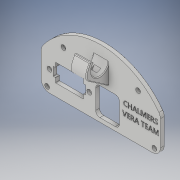
# Autodesk Inventor part: AdapterChassiContact
Saved by Autodesk Inventor 2019.3 (Build 233278000, 278)
## iProperties
Created: 2019-02-24
Part Number: AdapterChassiContact
Material: Generic
Document SubType Name: Modeling
Designer: Johansson
Density: 1 g/cm^3
Appearance: Default
Author: Johansson
## iProperties of the stored document AdapterChassiContact_3DPrint.ipt
Created: 2019-02-24
Part Number: AdapterChassiContact_3DPrint
Material: Generic
Document SubType Name: Modeling
Designer: Johansson
Density: 1 g/cm^3
Appearance: Default
Author: Johansson
Autodesk Inventor part; units mm, degrees
(part 1 of 4)
ref_plane "YZ Plane" through (0, 0, 0) normal (1, 0, 0) x (0, 1, 0)
ref_plane "XZ Plane" through (0, 0, 0) normal (0, 1, 0) x (-1, 0, 0)
ref_plane "XY Plane" through (0, 0, 0) normal (0, 0, 1) x (1, 0, 0)
sketch "Sketch1" plane through (0, 0, 0) normal (0, 0, 1) x (1, 0, 0)
  line L0 (-75, -22.5) -> (75, -22.5)
  line L1 (75, -22.5) -> (75, 22.5)
  line L2 (75, 22.5) -> (-75, 22.5)
  line L3 (-75, 22.5) -> (-75, -22.5)
  line L4 (-75, -22.5) -> (75, 22.5) construction
  line L5 (75, -22.5) -> (-75, 22.5) construction
  arc A0 (75, 22.5) -> (-75, 22.5) centre (0, -27.8125) ccw
  point P0 (0, 0)
  dimension "d0" = 150
  dimension "d1" = 85
  dimension "d2" = 45
  constraints: 12 end point, 2 midpoint, 2 parallel, 2 point on circle, 1 centre point, 1 horizontal, 1 perpendicular
  measures "d0" distance of L0.start L0.end
  measures "d1" distance edge to line of A0 L0
  measures "d2" distance of L0.end L1.end
extrude "Extrusion1" add sketch "Sketch1" along normal blind 5
sketch "Sketch2" plane through (0, 0, 5) normal (0, 0, 1) x (1, 0, 0)
  spline S0 degree 3 poles (-2.5291, 34.9419) (-3.1837, 35.0019) (-3.8439, 35.3955) (-4.2067, 35.9422) knots 0 0 0 0 1 1 1 1
  line L0 (-2.5291, 34.9419) -> (-3.1837, 35.0019) construction
  line L1 (-3.1837, 35.0019) -> (-3.8439, 35.3955) construction
  line L2 (-3.8439, 35.3955) -> (-4.2067, 35.9422) construction
  spline S1 degree 3 poles (-4.2067, 35.9422) (-4.5423, 36.4477) (-4.6869, 37.074) (-4.5949, 37.6226) knots 1 1 1 1 2 2 2 2
  line L3 (-4.2067, 35.9422) -> (-4.5423, 36.4477) construction
  line L4 (-4.5423, 36.4477) -> (-4.6869, 37.074) construction
  line L5 (-4.6869, 37.074) -> (-4.5949, 37.6226) construction
  spline S2 degree 3 poles (-4.5949, 37.6226) (-4.5028, 38.1713) (-4.29, 38.5913) (-3.9153, 38.9637) knots 2 2 2 2 3 3 3 3
  line L6 (-4.5949, 37.6226) -> (-4.5028, 38.1713) construction
  line L7 (-4.5028, 38.1713) -> (-4.29, 38.5913) construction
  line L8 (-4.29, 38.5913) -> (-3.9153, 38.9637) construction
  spline S3 degree 3 poles (-3.9153, 38.9637) (-3.6201, 39.257) (-3.2509, 39.4631) (-2.8284, 39.5702) knots 3 3 3 3 4 4 4 4
  line L9 (-3.9153, 38.9637) -> (-3.6201, 39.257) construction
  line L10 (-3.6201, 39.257) -> (-3.2509, 39.4631) construction
  line L11 (-3.2509, 39.4631) -> (-2.8284, 39.5702) construction
  spline S4 degree 3 poles (-2.8284, 39.5702) (-2.5997, 39.6282) (-2.3286, 39.6529) (-2.1379, 39.6331) knots 4 4 4 4 5 5 5 5
  line L12 (-2.8284, 39.5702) -> (-2.5997, 39.6282) construction
  line L13 (-2.5997, 39.6282) -> (-2.3286, 39.6529) construction
  line L14 (-2.3286, 39.6529) -> (-2.1379, 39.6331) construction
  spline S5 degree 3 poles (-2.1379, 39.6331) (-1.8898, 39.6073) (-1.8541, 39.6014) (-1.7115, 39.563) knots 5 5 5 5 6 6 6 6
  line L15 (-2.1379, 39.6331) -> (-1.8898, 39.6073) construction
  line L16 (-1.8898, 39.6073) -> (-1.8541, 39.6014) construction
  line L17 (-1.8541, 39.6014) -> (-1.7115, 39.563) construction
  spline S6 degree 3 poles (-1.7115, 39.563) (-1.5406, 39.517) (-1.5075, 39.5031) (-0.386, 39.0072) knots 6 6 6 6 7 7 7 7
  line L18 (-1.7115, 39.563) -> (-1.5406, 39.517) construction
  line L19 (-1.5406, 39.517) -> (-1.5075, 39.5031) construction
  line L20 (-1.5075, 39.5031) -> (-0.386, 39.0072) construction
  spline S7 degree 3 poles (-0.386, 39.0072) (0.5004, 38.6152) (0.8357, 38.4674) (0.9545, 38.4164) knots 7 7 7 7 8 8 8 8
  line L21 (-0.386, 39.0072) -> (0.5004, 38.6152) construction
  line L22 (0.5004, 38.6152) -> (0.8357, 38.4674) construction
  line L23 (0.8357, 38.4674) -> (0.9545, 38.4164) construction
  spline S8 degree 3 poles (0.9545, 38.4164) (1.1108, 38.3493) (1.1389, 38.3282) (1.072, 38.3282) (1.0454, 38.3282) (0.9942, 38.3132) (0.9582, 38.2948) knots 8 8 8 8 9 9 9 10 10 10 10
  line L24 (0.9545, 38.4164) -> (1.1108, 38.3493) construction
  line L25 (1.1108, 38.3493) -> (1.1389, 38.3282) construction
  line L26 (1.1389, 38.3282) -> (1.072, 38.3282) construction
  line L27 (1.072, 38.3282) -> (1.0454, 38.3282) construction
  line L28 (1.0454, 38.3282) -> (0.9942, 38.3132) construction
  line L29 (0.9942, 38.3132) -> (0.9582, 38.2948) construction
  line L30 (0.9582, 38.2948) -> (0.8926, 38.2613)
  line L31 (0.8926, 38.2613) -> (0.2754, 38.5244)
  spline S9 degree 3 poles (0.2754, 38.5244) (-0.0641, 38.6691) (-0.4798, 38.8468) (-0.6484, 38.9191) (-0.817, 38.9915) (-0.9608, 39.0471) (-0.968, 39.0426) knots 12 12 12 12 13 13 13 14 14 14 14
  line L32 (0.2754, 38.5244) -> (-0.0641, 38.6691) construction
  line L33 (-0.0641, 38.6691) -> (-0.4798, 38.8468) construction
  line L34 (-0.4798, 38.8468) -> (-0.6484, 38.9191) construction
  line L35 (-0.6484, 38.9191) -> (-0.817, 38.9915) construction
  line L36 (-0.817, 38.9915) -> (-0.9608, 39.0471) construction
  line L37 (-0.9608, 39.0471) -> (-0.968, 39.0426) construction
  spline S10 degree 3 poles (-0.968, 39.0426) (-0.9926, 39.0275) (-1.0039, 38.9233) (-0.9836, 38.899) knots 14 14 14 14 15 15 15 15
  line L38 (-0.968, 39.0426) -> (-0.9926, 39.0275) construction
  line L39 (-0.9926, 39.0275) -> (-1.0039, 38.9233) construction
  line L40 (-1.0039, 38.9233) -> (-0.9836, 38.899) construction
  spline S11 degree 3 poles (-0.9836, 38.899) (-0.9576, 38.8675) (-0.8953, 38.8685) (-0.8524, 38.9009) knots 15 15 15 15 16 16 16 16
  line L41 (-0.9836, 38.899) -> (-0.9576, 38.8675) construction
  line L42 (-0.9576, 38.8675) -> (-0.8953, 38.8685) construction
  line L43 (-0.8953, 38.8685) -> (-0.8524, 38.9009) construction
  spline S12 degree 3 poles (-0.8524, 38.9009) (-0.7927, 38.9461) (-0.7695, 38.935) (-0.8001, 38.8759) knots 16 16 16 16 17 17 17 17
  line L44 (-0.8524, 38.9009) -> (-0.7927, 38.9461) construction
  line L45 (-0.7927, 38.9461) -> (-0.7695, 38.935) construction
  line L46 (-0.7695, 38.935) -> (-0.8001, 38.8759) construction
  spline S13 degree 3 poles (-0.8001, 38.8759) (-0.8345, 38.8092) (-0.8342, 38.7619) (-0.7991, 38.7328) knots 17 17 17 17 18 18 18 18
  line L47 (-0.8001, 38.8759) -> (-0.8345, 38.8092) construction
  line L48 (-0.8345, 38.8092) -> (-0.8342, 38.7619) construction
  line L49 (-0.8342, 38.7619) -> (-0.7991, 38.7328) construction
  spline S14 degree 3 poles (-0.7991, 38.7328) (-0.7761, 38.7136) (-0.758, 38.7146) (-0.6933, 38.7386) knots 18 18 18 18 19 19 19 19
  line L50 (-0.7991, 38.7328) -> (-0.7761, 38.7136) construction
  line L51 (-0.7761, 38.7136) -> (-0.758, 38.7146) construction
  line L52 (-0.758, 38.7146) -> (-0.6933, 38.7386) construction
  spline S15 degree 3 poles (-0.6933, 38.7386) (-0.6055, 38.7711) (-0.6012, 38.766) (-0.6497, 38.6865) knots 19 19 19 19 20 20 20 20
  line L53 (-0.6933, 38.7386) -> (-0.6055, 38.7711) construction
  line L54 (-0.6055, 38.7711) -> (-0.6012, 38.766) construction
  line L55 (-0.6012, 38.766) -> (-0.6497, 38.6865) construction
  spline S16 degree 3 poles (-0.6497, 38.6865) (-0.6836, 38.6309) (-0.6836, 38.63) (-0.6495, 38.5866) knots 20 20 20 20 21 21 21 21
  line L56 (-0.6497, 38.6865) -> (-0.6836, 38.6309) construction
  line L57 (-0.6836, 38.6309) -> (-0.6836, 38.63) construction
  line L58 (-0.6836, 38.63) -> (-0.6495, 38.5866) construction
  spline S17 degree 3 poles (-0.6495, 38.5866) (-0.6157, 38.5436) (-0.6137, 38.5433) (-0.5444, 38.5706) knots 21 21 21 21 22 22 22 22
  line L59 (-0.6495, 38.5866) -> (-0.6157, 38.5436) construction
  line L60 (-0.6157, 38.5436) -> (-0.6137, 38.5433) construction
  line L61 (-0.6137, 38.5433) -> (-0.5444, 38.5706) construction
  spline S18 degree 3 poles (-0.5444, 38.5706) (-0.5056, 38.5858) (-0.4691, 38.5936) (-0.4634, 38.5879) knots 22 22 22 22 23 23 23 23
  line L62 (-0.5444, 38.5706) -> (-0.5056, 38.5858) construction
  line L63 (-0.5056, 38.5858) -> (-0.4691, 38.5936) construction
  line L64 (-0.4691, 38.5936) -> (-0.4634, 38.5879) construction
  spline S19 degree 3 poles (-0.4634, 38.5879) (-0.4577, 38.5822) (-0.4736, 38.5504) (-0.4989, 38.5173) knots 23 23 23 23 24 24 24 24
  line L65 (-0.4634, 38.5879) -> (-0.4577, 38.5822) construction
  line L66 (-0.4577, 38.5822) -> (-0.4736, 38.5504) construction
  line L67 (-0.4736, 38.5504) -> (-0.4989, 38.5173) construction
  spline S20 degree 3 poles (-0.4989, 38.5173) (-0.552, 38.4477) (-0.5549, 38.4291) (-0.5176, 38.3982) knots 24 24 24 24 25 25 25 25
  line L68 (-0.4989, 38.5173) -> (-0.552, 38.4477) construction
  line L69 (-0.552, 38.4477) -> (-0.5549, 38.4291) construction
  line L70 (-0.5549, 38.4291) -> (-0.5176, 38.3982) construction
  spline S21 degree 3 poles (-0.5176, 38.3982) (-0.4964, 38.3806) (-0.476, 38.3801) (-0.4254, 38.3956) knots 25 25 25 25 26 26 26 26
  line L71 (-0.5176, 38.3982) -> (-0.4964, 38.3806) construction
  line L72 (-0.4964, 38.3806) -> (-0.476, 38.3801) construction
  line L73 (-0.476, 38.3801) -> (-0.4254, 38.3956) construction
  spline S22 degree 3 poles (-0.4254, 38.3956) (-0.3345, 38.4235) (-0.3128, 38.3954) (-0.3752, 38.3302) knots 26 26 26 26 27 27 27 27
  line L74 (-0.4254, 38.3956) -> (-0.3345, 38.4235) construction
  line L75 (-0.3345, 38.4235) -> (-0.3128, 38.3954) construction
  line L76 (-0.3128, 38.3954) -> (-0.3752, 38.3302) construction
  spline S23 degree 3 poles (-0.3752, 38.3302) (-0.4071, 38.297) (-0.4222, 38.2646) (-0.4183, 38.2375) knots 27 27 27 27 28 28 28 28
  line L77 (-0.3752, 38.3302) -> (-0.4071, 38.297) construction
  line L78 (-0.4071, 38.297) -> (-0.4222, 38.2646) construction
  line L79 (-0.4222, 38.2646) -> (-0.4183, 38.2375) construction
  spline S24 degree 3 poles (-0.4183, 38.2375) (-0.4129, 38.199) (-0.4056, 38.1963) (-0.3198, 38.2016) knots 28 28 28 28 29 29 29 29
  line L80 (-0.4183, 38.2375) -> (-0.4129, 38.199) construction
  line L81 (-0.4129, 38.199) -> (-0.4056, 38.1963) construction
  line L82 (-0.4056, 38.1963) -> (-0.3198, 38.2016) construction
  spline S25 degree 3 poles (-0.3198, 38.2016) (-0.2689, 38.2047) (-0.2272, 38.2011) (-0.2272, 38.1936) (-0.2272, 38.1861) (-0.2524, 38.154) (-0.2832, 38.1222) knots 29 29 29 29 30 30 30 31 31 31 31
  line L83 (-0.3198, 38.2016) -> (-0.2689, 38.2047) construction
  line L84 (-0.2689, 38.2047) -> (-0.2272, 38.2011) construction
  line L85 (-0.2272, 38.2011) -> (-0.2272, 38.1936) construction
  line L86 (-0.2272, 38.1936) -> (-0.2272, 38.1861) construction
  line L87 (-0.2272, 38.1861) -> (-0.2524, 38.154) construction
  line L88 (-0.2524, 38.154) -> (-0.2832, 38.1222) construction
  spline S26 degree 3 poles (-0.2832, 38.1222) (-0.333, 38.0708) (-0.3369, 38.0596) (-0.3188, 38.02) knots 31 31 31 31 32 32 32 32
  line L89 (-0.2832, 38.1222) -> (-0.333, 38.0708) construction
  line L90 (-0.333, 38.0708) -> (-0.3369, 38.0596) construction
  line L91 (-0.3369, 38.0596) -> (-0.3188, 38.02) construction
  spline S27 degree 3 poles (-0.3188, 38.02) (-0.3014, 37.9816) (-0.287, 37.9753) (-0.2144, 37.9748) knots 32 32 32 32 33 33 33 33
  line L92 (-0.3188, 38.02) -> (-0.3014, 37.9816) construction
  line L93 (-0.3014, 37.9816) -> (-0.287, 37.9753) construction
  line L94 (-0.287, 37.9753) -> (-0.2144, 37.9748) construction
  line L95 (-0.2144, 37.9748) -> (-0.1302, 37.9741)
  line L96 (-0.1302, 37.9741) -> (-0.1964, 37.9174)
  spline S28 degree 3 poles (-0.1964, 37.9174) (-0.2328, 37.8863) (-0.2625, 37.8472) (-0.2625, 37.8305) (-0.2625, 37.7908) (-0.2095, 37.7638) (-0.1314, 37.7638) (-0.0518, 37.7638) (-0.0515, 37.742) (-0.1307, 37.6953) knots 35 35 35 35 36 36 36 37 37 37 38 38 38 38
  line L97 (-0.1964, 37.9174) -> (-0.2328, 37.8863) construction
  line L98 (-0.2328, 37.8863) -> (-0.2625, 37.8472) construction
  line L99 (-0.2625, 37.8472) -> (-0.2625, 37.8305) construction
  line L100 (-0.2625, 37.8305) -> (-0.2625, 37.7908) construction
  line L101 (-0.2625, 37.7908) -> (-0.2095, 37.7638) construction
  line L102 (-0.2095, 37.7638) -> (-0.1314, 37.7638) construction
  line L103 (-0.1314, 37.7638) -> (-0.0518, 37.7638) construction
  line L104 (-0.0518, 37.7638) -> (-0.0515, 37.742) construction
  line L105 (-0.0515, 37.742) -> (-0.1307, 37.6953) construction
  spline S29 degree 3 poles (-0.1307, 37.6953) (-0.2375, 37.6322) (-0.2296, 37.5664) (-0.1126, 37.5444) knots 38 38 38 38 39 39 39 39
  line L106 (-0.1307, 37.6953) -> (-0.2375, 37.6322) construction
  line L107 (-0.2375, 37.6322) -> (-0.2296, 37.5664) construction
  line L108 (-0.2296, 37.5664) -> (-0.1126, 37.5444) construction
  spline S30 degree 3 poles (-0.1126, 37.5444) (-0.025, 37.528) (-0.0224, 37.5054) (-0.1032, 37.4642) knots 39 39 39 39 40 40 40 40
  line L109 (-0.1126, 37.5444) -> (-0.025, 37.528) construction
  line L110 (-0.025, 37.528) -> (-0.0224, 37.5054) construction
  line L111 (-0.0224, 37.5054) -> (-0.1032, 37.4642) construction
  spline S31 degree 3 poles (-0.1032, 37.4642) (-0.1559, 37.4373) (-0.1743, 37.4171) (-0.1743, 37.3863) (-0.1743, 37.3358) (-0.1496, 37.3136) (-0.0685, 37.2914) knots 40 40 40 40 41 41 41 42 42 42 42
  line L112 (-0.1032, 37.4642) -> (-0.1559, 37.4373) construction
  line L113 (-0.1559, 37.4373) -> (-0.1743, 37.4171) construction
  line L114 (-0.1743, 37.4171) -> (-0.1743, 37.3863) construction
  line L115 (-0.1743, 37.3863) -> (-0.1743, 37.3358) construction
  line L116 (-0.1743, 37.3358) -> (-0.1496, 37.3136) construction
  line L117 (-0.1496, 37.3136) -> (-0.0685, 37.2914) construction
  line L118 (-0.0685, 37.2914) -> (-0.0068, 37.2745)
  line L119 (-0.0068, 37.2745) -> (-0.0597, 37.2545)
  spline S32 degree 3 poles (-0.0597, 37.2545) (-0.1458, 37.2221) (-0.1652, 37.2067) (-0.1713, 37.1657) knots 44 44 44 44 45 45 45 45
  line L120 (-0.0597, 37.2545) -> (-0.1458, 37.2221) construction
  line L121 (-0.1458, 37.2221) -> (-0.1652, 37.2067) construction
  line L122 (-0.1652, 37.2067) -> (-0.1713, 37.1657) construction
  spline S33 degree 3 poles (-0.1713, 37.1657) (-0.1788, 37.115) (-0.149, 37.0808) (-0.0849, 37.0668) knots 45 45 45 45 46 46 46 46
  line L123 (-0.1713, 37.1657) -> (-0.1788, 37.115) construction
  line L124 (-0.1788, 37.115) -> (-0.149, 37.0808) construction
  line L125 (-0.149, 37.0808) -> (-0.0849, 37.0668) construction
  spline S34 degree 3 poles (-0.0849, 37.0668) (-0.0168, 37.0518) (-0.0193, 37.0287) (-0.0905, 37.0135) knots 46 46 46 46 47 47 47 47
  line L126 (-0.0849, 37.0668) -> (-0.0168, 37.0518) construction
  line L127 (-0.0168, 37.0518) -> (-0.0193, 37.0287) construction
  line L128 (-0.0193, 37.0287) -> (-0.0905, 37.0135) construction
  spline S35 degree 3 poles (-0.0905, 37.0135) (-0.1665, 36.9972) (-0.192, 36.9746) (-0.192, 36.9232) (-0.192, 36.8928) (-0.1732, 36.8696) (-0.1264, 36.8419) knots 47 47 47 47 48 48 48 49 49 49 49
  line L129 (-0.0905, 37.0135) -> (-0.1665, 36.9972) construction
  line L130 (-0.1665, 36.9972) -> (-0.192, 36.9746) construction
  line L131 (-0.192, 36.9746) -> (-0.192, 36.9232) construction
  line L132 (-0.192, 36.9232) -> (-0.192, 36.8928) construction
  line L133 (-0.192, 36.8928) -> (-0.1732, 36.8696) construction
  line L134 (-0.1732, 36.8696) -> (-0.1264, 36.8419) construction
  line L135 (-0.1264, 36.8419) -> (-0.0608, 36.8032)
  line L136 (-0.0608, 36.8032) -> (-0.1355, 36.7905)
  spline S36 degree 3 poles (-0.1355, 36.7905) (-0.2322, 36.774) (-0.2449, 36.765) (-0.2449, 36.7134) (-0.2449, 36.6838) (-0.2258, 36.6581) (-0.1834, 36.6306) knots 51 51 51 51 52 52 52 53 53 53 53
  line L137 (-0.1355, 36.7905) -> (-0.2322, 36.774) construction
  line L138 (-0.2322, 36.774) -> (-0.2449, 36.765) construction
  line L139 (-0.2449, 36.765) -> (-0.2449, 36.7134) construction
  line L140 (-0.2449, 36.7134) -> (-0.2449, 36.6838) construction
  line L141 (-0.2449, 36.6838) -> (-0.2258, 36.6581) construction
  line L142 (-0.2258, 36.6581) -> (-0.1834, 36.6306) construction
  spline S37 degree 3 poles (-0.1834, 36.6306) (-0.1495, 36.6087) (-0.1218, 36.5848) (-0.1216, 36.5775) knots 53 53 53 53 54 54 54 54
  line L143 (-0.1834, 36.6306) -> (-0.1495, 36.6087) construction
  line L144 (-0.1495, 36.6087) -> (-0.1218, 36.5848) construction
  line L145 (-0.1218, 36.5848) -> (-0.1216, 36.5775) construction
  spline S38 degree 3 poles (-0.1216, 36.5775) (-0.1215, 36.5703) (-0.1573, 36.5643) (-0.2012, 36.5643) (-0.2693, 36.5643) (-0.2839, 36.5578) (-0.3012, 36.5198) knots 54 54 54 54 55 55 55 56 56 56 56
  line L146 (-0.1216, 36.5775) -> (-0.1215, 36.5703) construction
  line L147 (-0.1215, 36.5703) -> (-0.1573, 36.5643) construction
  line L148 (-0.1573, 36.5643) -> (-0.2012, 36.5643) construction
  line L149 (-0.2012, 36.5643) -> (-0.2693, 36.5643) construction
  line L150 (-0.2693, 36.5643) -> (-0.2839, 36.5578) construction
  line L151 (-0.2839, 36.5578) -> (-0.3012, 36.5198) construction
  spline S39 degree 3 poles (-0.3012, 36.5198) (-0.3194, 36.4799) (-0.3153, 36.4688) (-0.2621, 36.414) knots 56 56 56 56 57 57 57 57
  line L152 (-0.3012, 36.5198) -> (-0.3194, 36.4799) construction
  line L153 (-0.3194, 36.4799) -> (-0.3153, 36.4688) construction
  line L154 (-0.3153, 36.4688) -> (-0.2621, 36.414) construction
  line L155 (-0.2621, 36.414) -> (-0.2027, 36.3526)
  line L156 (-0.2027, 36.3526) -> (-0.282, 36.3526)
  spline S40 degree 3 poles (-0.282, 36.3526) (-0.4153, 36.3526) (-0.4392, 36.2947) (-0.3463, 36.1971) knots 59 59 59 59 60 60 60 60
  line L157 (-0.282, 36.3526) -> (-0.4153, 36.3526) construction
  line L158 (-0.4153, 36.3526) -> (-0.4392, 36.2947) construction
  line L159 (-0.4392, 36.2947) -> (-0.3463, 36.1971) construction
  line L160 (-0.3463, 36.1971) -> (-0.289, 36.1368)
  line L161 (-0.289, 36.1368) -> (-0.3739, 36.1489)
  spline S41 degree 3 poles (-0.3739, 36.1489) (-0.5046, 36.1677) (-0.5488, 36.1076) (-0.4742, 36.0127) knots 62 62 62 62 63 63 63 63
  line L162 (-0.3739, 36.1489) -> (-0.5046, 36.1677) construction
  line L163 (-0.5046, 36.1677) -> (-0.5488, 36.1076) construction
  line L164 (-0.5488, 36.1076) -> (-0.4742, 36.0127) construction
  spline S42 degree 3 poles (-0.4742, 36.0127) (-0.4548, 35.988) (-0.4389, 35.9623) (-0.4389, 35.9555) (-0.4389, 35.9436) (-0.4945, 35.9532) (-0.5506, 35.9747) knots 63 63 63 63 64 64 64 65 65 65 65
  line L165 (-0.4742, 36.0127) -> (-0.4548, 35.988) construction
  line L166 (-0.4548, 35.988) -> (-0.4389, 35.9623) construction
  line L167 (-0.4389, 35.9623) -> (-0.4389, 35.9555) construction
  line L168 (-0.4389, 35.9555) -> (-0.4389, 35.9436) construction
  line L169 (-0.4389, 35.9436) -> (-0.4945, 35.9532) construction
  line L170 (-0.4945, 35.9532) -> (-0.5506, 35.9747) construction
  spline S43 degree 3 poles (-0.5506, 35.9747) (-0.5654, 35.9804) (-0.5937, 35.9686) (-0.6142, 35.9481) knots 65 65 65 65 66 66 66 66
  line L171 (-0.5506, 35.9747) -> (-0.5654, 35.9804) construction
  line L172 (-0.5654, 35.9804) -> (-0.5937, 35.9686) construction
  line L173 (-0.5937, 35.9686) -> (-0.6142, 35.9481) construction
  line L174 (-0.6142, 35.9481) -> (-0.6511, 35.9112)
  line L175 (-0.6511, 35.9112) -> (-0.6155, 35.8416)
  spline S44 degree 3 poles (-0.6155, 35.8416) (-0.5691, 35.7506) (-0.5702, 35.7469) (-0.6341, 35.78) knots 68 68 68 68 69 69 69 69
  line L176 (-0.6155, 35.8416) -> (-0.5691, 35.7506) construction
  line L177 (-0.5691, 35.7506) -> (-0.5702, 35.7469) construction
  line L178 (-0.5702, 35.7469) -> (-0.6341, 35.78) construction
  spline S45 degree 3 poles (-0.6341, 35.78) (-0.6987, 35.8134) (-0.7546, 35.8083) (-0.7807, 35.7666) knots 69 69 69 69 70 70 70 70
  line L179 (-0.6341, 35.78) -> (-0.6987, 35.8134) construction
  line L180 (-0.6987, 35.8134) -> (-0.7546, 35.8083) construction
  line L181 (-0.7546, 35.8083) -> (-0.7807, 35.7666) construction
  spline S46 degree 3 poles (-0.7807, 35.7666) (-0.7994, 35.7368) (-0.7973, 35.7265) (-0.7466, 35.604) knots 70 70 70 70 71 71 71 71
  line L182 (-0.7807, 35.7666) -> (-0.7994, 35.7368) construction
  line L183 (-0.7994, 35.7368) -> (-0.7973, 35.7265) construction
  line L184 (-0.7973, 35.7265) -> (-0.7466, 35.604) construction
  spline S47 degree 3 poles (-0.7466, 35.604) (-0.7333, 35.572) (-0.7367, 35.5724) (-0.797, 35.6097) knots 71 71 71 71 72 72 72 72
  line L185 (-0.7466, 35.604) -> (-0.7333, 35.572) construction
  line L186 (-0.7333, 35.572) -> (-0.7367, 35.5724) construction
  line L187 (-0.7367, 35.5724) -> (-0.797, 35.6097) construction
  spline S48 degree 3 poles (-0.797, 35.6097) (-0.889, 35.6665) (-0.9404, 35.6551) (-0.9462, 35.5765) knots 72 72 72 72 73 73 73 73
  line L188 (-0.797, 35.6097) -> (-0.889, 35.6665) construction
  line L189 (-0.889, 35.6665) -> (-0.9404, 35.6551) construction
  line L190 (-0.9404, 35.6551) -> (-0.9462, 35.5765) construction
  spline S49 degree 3 poles (-0.9462, 35.5765) (-0.9554, 35.4536) (-0.9433, 35.4538) (-0.6443, 35.5823) knots 73 73 73 73 74 74 74 74
  line L191 (-0.9462, 35.5765) -> (-0.9554, 35.4536) construction
  line L192 (-0.9554, 35.4536) -> (-0.9433, 35.4538) construction
  line L193 (-0.9433, 35.4538) -> (-0.6443, 35.5823) construction
  spline S50 degree 3 poles (-0.6443, 35.5823) (-0.4937, 35.647) (-0.3654, 35.7) (-0.3592, 35.7) (-0.353, 35.7) (-0.2196, 35.7549) (-0.0627, 35.8219) knots 74 74 74 74 75 75 75 76 76 76 76
  line L194 (-0.6443, 35.5823) -> (-0.4937, 35.647) construction
  line L195 (-0.4937, 35.647) -> (-0.3654, 35.7) construction
  line L196 (-0.3654, 35.7) -> (-0.3592, 35.7) construction
  line L197 (-0.3592, 35.7) -> (-0.353, 35.7) construction
  line L198 (-0.353, 35.7) -> (-0.2196, 35.7549) construction
  line L199 (-0.2196, 35.7549) -> (-0.0627, 35.8219) construction
  spline S51 degree 3 poles (-0.0627, 35.8219) (0.0942, 35.889) (0.337, 35.9927) (0.4769, 36.0523) knots 76 76 76 76 77 77 77 77
  line L200 (-0.0627, 35.8219) -> (0.0942, 35.889) construction
  line L201 (0.0942, 35.889) -> (0.337, 35.9927) construction
  line L202 (0.337, 35.9927) -> (0.4769, 36.0523) construction
  spline S52 degree 3 poles (0.4769, 36.0523) (0.6168, 36.112) (0.7546, 36.1729) (0.783, 36.1876) knots 77 77 77 77 78 78 78 78
  line L203 (0.4769, 36.0523) -> (0.6168, 36.112) construction
  line L204 (0.6168, 36.112) -> (0.7546, 36.1729) construction
  line L205 (0.7546, 36.1729) -> (0.783, 36.1876) construction
  spline S53 degree 3 poles (0.783, 36.1876) (0.833, 36.2134) (0.8367, 36.2125) (0.8866, 36.1615) knots 78 78 78 78 79 79 79 79
  line L206 (0.783, 36.1876) -> (0.833, 36.2134) construction
  line L207 (0.833, 36.2134) -> (0.8367, 36.2125) construction
  line L208 (0.8367, 36.2125) -> (0.8866, 36.1615) construction
  spline S54 degree 3 poles (0.8866, 36.1615) (0.915, 36.1324) (0.932, 36.1049) (0.9244, 36.1003) knots 79 79 79 79 80 80 80 80
  line L209 (0.8866, 36.1615) -> (0.915, 36.1324) construction
  line L210 (0.915, 36.1324) -> (0.932, 36.1049) construction
  line L211 (0.932, 36.1049) -> (0.9244, 36.1003) construction
  spline S55 degree 3 poles (0.9244, 36.1003) (0.9167, 36.0958) (0.7795, 36.0389) (0.6194, 35.9738) knots 80 80 80 80 81 81 81 81
  line L212 (0.9244, 36.1003) -> (0.9167, 36.0958) construction
  line L213 (0.9167, 36.0958) -> (0.7795, 36.0389) construction
  line L214 (0.7795, 36.0389) -> (0.6194, 35.9738) construction
  spline S56 degree 3 poles (0.6194, 35.9738) (0.4593, 35.9087) (0.3204, 35.8495) (0.3107, 35.8422) knots 81 81 81 81 82 82 82 82
  line L215 (0.6194, 35.9738) -> (0.4593, 35.9087) construction
  line L216 (0.4593, 35.9087) -> (0.3204, 35.8495) construction
  line L217 (0.3204, 35.8495) -> (0.3107, 35.8422) construction
  spline S57 degree 3 poles (0.3107, 35.8422) (0.301, 35.8348) (0.2296, 35.8028) (0.152, 35.7711) knots 82 82 82 82 83 83 83 83
  line L218 (0.3107, 35.8422) -> (0.301, 35.8348) construction
  line L219 (0.301, 35.8348) -> (0.2296, 35.8028) construction
  line L220 (0.2296, 35.8028) -> (0.152, 35.7711) construction
  spline S58 degree 3 poles (0.152, 35.7711) (0.0744, 35.7394) (-0.0883, 35.6716) (-0.2096, 35.6205) (-0.3309, 35.5694) (-0.5746, 35.4669) (-0.7512, 35.3928) knots 83 83 83 83 84 84 84 85 85 85 85
  line L221 (0.152, 35.7711) -> (0.0744, 35.7394) construction
  line L222 (0.0744, 35.7394) -> (-0.0883, 35.6716) construction
  line L223 (-0.0883, 35.6716) -> (-0.2096, 35.6205) construction
  line L224 (-0.2096, 35.6205) -> (-0.3309, 35.5694) construction
  line L225 (-0.3309, 35.5694) -> (-0.5746, 35.4669) construction
  line L226 (-0.5746, 35.4669) -> (-0.7512, 35.3928) construction
  spline S59 degree 3 poles (-0.7512, 35.3928) (-0.9278, 35.3187) (-1.1563, 35.2189) (-1.259, 35.1709) knots 85 85 85 85 86 86 86 86
  line L227 (-0.7512, 35.3928) -> (-0.9278, 35.3187) construction
  line L228 (-0.9278, 35.3187) -> (-1.1563, 35.2189) construction
  line L229 (-1.1563, 35.2189) -> (-1.259, 35.1709) construction
  spline S60 degree 3 poles (-1.259, 35.1709) (-1.6777, 34.9754) (-2.0878, 34.9015) (-2.5291, 34.9419) knots 86 86 86 86 87 87 87 87
  line L230 (-1.259, 35.1709) -> (-1.6777, 34.9754) construction
  line L231 (-1.6777, 34.9754) -> (-2.0878, 34.9015) construction
  line L232 (-2.0878, 34.9015) -> (-2.5291, 34.9419) construction
  line L233 (-2.5291, 34.9419) -> (-2.5291, 34.9419)
  spline S61 degree 3 poles (-2.291, 35.0968) (-2.291, 35.121) (-2.332, 35.1532) (-2.3629, 35.1532) (-2.397, 35.1532) (-2.4375, 35.1115) (-2.4202, 35.0943) (-2.4036, 35.0777) (-2.291, 35.0799) (-2.291, 35.0968) knots 0 0 0 0 1 1 1 2 2 2 3 3 3 3
  line L234 (-2.291, 35.0968) -> (-2.291, 35.121) construction
  line L235 (-2.291, 35.121) -> (-2.332, 35.1532) construction
  line L236 (-2.332, 35.1532) -> (-2.3629, 35.1532) construction
  line L237 (-2.3629, 35.1532) -> (-2.397, 35.1532) construction
  line L238 (-2.397, 35.1532) -> (-2.4375, 35.1115) construction
  line L239 (-2.4375, 35.1115) -> (-2.4202, 35.0943) construction
  line L240 (-2.4202, 35.0943) -> (-2.4036, 35.0777) construction
  line L241 (-2.4036, 35.0777) -> (-2.291, 35.0799) construction
  line L242 (-2.291, 35.0799) -> (-2.291, 35.0968) construction
  spline S62 degree 3 poles (-2.0657, 35.1034) (-2.0786, 35.1423) (-2.1299, 35.1634) (-2.1621, 35.143) (-2.2203, 35.1063) (-2.2086, 35.0826) (-2.1323, 35.0826) (-2.0837, 35.0826) (-2.0611, 35.0897) (-2.0657, 35.1034) knots 0 0 0 0 1 1 1 2 2 2 3 3 3 3
  line L243 (-2.0657, 35.1034) -> (-2.0786, 35.1423) construction
  line L244 (-2.0786, 35.1423) -> (-2.1299, 35.1634) construction
  line L245 (-2.1299, 35.1634) -> (-2.1621, 35.143) construction
  line L246 (-2.1621, 35.143) -> (-2.2203, 35.1063) construction
  line L247 (-2.2203, 35.1063) -> (-2.2086, 35.0826) construction
  line L248 (-2.2086, 35.0826) -> (-2.1323, 35.0826) construction
  line L249 (-2.1323, 35.0826) -> (-2.0837, 35.0826) construction
  line L250 (-2.0837, 35.0826) -> (-2.0611, 35.0897) construction
  line L251 (-2.0611, 35.0897) -> (-2.0657, 35.1034) construction
  spline S63 degree 3 poles (-2.5147, 35.1267) (-2.5165, 35.1364) (-2.5329, 35.1543) (-2.5511, 35.1664) (-2.5778, 35.1841) (-2.5905, 35.1838) (-2.6167, 35.1647) (-2.6355, 35.1509) (-2.6436, 35.132) (-2.636, 35.1196) (-2.6205, 35.0945) (-2.51, 35.101) (-2.5147, 35.1267) knots 0 0 0 0 1 1 1 2 2 2 3 3 3 4 4 4 4
  line L252 (-2.5147, 35.1267) -> (-2.5165, 35.1364) construction
  line L253 (-2.5165, 35.1364) -> (-2.5329, 35.1543) construction
  line L254 (-2.5329, 35.1543) -> (-2.5511, 35.1664) construction
  line L255 (-2.5511, 35.1664) -> (-2.5778, 35.1841) construction
  line L256 (-2.5778, 35.1841) -> (-2.5905, 35.1838) construction
  line L257 (-2.5905, 35.1838) -> (-2.6167, 35.1647) construction
  line L258 (-2.6167, 35.1647) -> (-2.6355, 35.1509) construction
  line L259 (-2.6355, 35.1509) -> (-2.6436, 35.132) construction
  line L260 (-2.6436, 35.132) -> (-2.636, 35.1196) construction
  line L261 (-2.636, 35.1196) -> (-2.6205, 35.0945) construction
  line L262 (-2.6205, 35.0945) -> (-2.51, 35.101) construction
  line L263 (-2.51, 35.101) -> (-2.5147, 35.1267) construction
  spline S64 degree 3 poles (-1.8336, 35.1286) (-1.8148, 35.1471) (-1.8681, 35.1731) (-1.9139, 35.1678) (-1.9465, 35.1641) (-1.9666, 35.1503) (-1.9707, 35.1289) (-1.9763, 35.0994) (-1.9694, 35.0971) (-1.9091, 35.1084) (-1.8718, 35.1154) (-1.8378, 35.1245) (-1.8336, 35.1286) knots 0 0 0 0 1 1 1 2 2 2 3 3 3 4 4 4 4
  line L264 (-1.8336, 35.1286) -> (-1.8148, 35.1471) construction
  line L265 (-1.8148, 35.1471) -> (-1.8681, 35.1731) construction
  line L266 (-1.8681, 35.1731) -> (-1.9139, 35.1678) construction
  line L267 (-1.9139, 35.1678) -> (-1.9465, 35.1641) construction
  line L268 (-1.9465, 35.1641) -> (-1.9666, 35.1503) construction
  line L269 (-1.9666, 35.1503) -> (-1.9707, 35.1289) construction
  line L270 (-1.9707, 35.1289) -> (-1.9763, 35.0994) construction
  line L271 (-1.9763, 35.0994) -> (-1.9694, 35.0971) construction
  line L272 (-1.9694, 35.0971) -> (-1.9091, 35.1084) construction
  line L273 (-1.9091, 35.1084) -> (-1.8718, 35.1154) construction
  line L274 (-1.8718, 35.1154) -> (-1.8378, 35.1245) construction
  line L275 (-1.8378, 35.1245) -> (-1.8336, 35.1286) construction
  spline S65 degree 3 poles (-2.732, 35.1624) (-2.732, 35.1772) (-2.7521, 35.1984) (-2.7767, 35.2096) (-2.8134, 35.2264) (-2.8267, 35.2248) (-2.8505, 35.201) (-2.8773, 35.1742) (-2.8763, 35.1708) (-2.8366, 35.1549) (-2.7726, 35.1294) (-2.732, 35.1323) (-2.732, 35.1624) knots 0 0 0 0 1 1 1 2 2 2 3 3 3 4 4 4 4
  line L276 (-2.732, 35.1624) -> (-2.732, 35.1772) construction
  line L277 (-2.732, 35.1772) -> (-2.7521, 35.1984) construction
  line L278 (-2.7521, 35.1984) -> (-2.7767, 35.2096) construction
  line L279 (-2.7767, 35.2096) -> (-2.8134, 35.2264) construction
  line L280 (-2.8134, 35.2264) -> (-2.8267, 35.2248) construction
  line L281 (-2.8267, 35.2248) -> (-2.8505, 35.201) construction
  line L282 (-2.8505, 35.201) -> (-2.8773, 35.1742) construction
  line L283 (-2.8773, 35.1742) -> (-2.8763, 35.1708) construction
  line L284 (-2.8763, 35.1708) -> (-2.8366, 35.1549) construction
  line L285 (-2.8366, 35.1549) -> (-2.7726, 35.1294) construction
  line L286 (-2.7726, 35.1294) -> (-2.732, 35.1323) construction
  line L287 (-2.732, 35.1323) -> (-2.732, 35.1624) construction
  spline S66 degree 3 poles (-1.6755, 35.1552) (-1.6168, 35.1757) (-1.6118, 35.1999) (-1.66, 35.2303) (-1.6953, 35.2526) (-1.7442, 35.2168) (-1.7442, 35.1687) (-1.7442, 35.1297) (-1.7471, 35.1302) (-1.6755, 35.1552) knots 0 0 0 0 1 1 1 2 2 2 3 3 3 3
  line L288 (-1.6755, 35.1552) -> (-1.6168, 35.1757) construction
  line L289 (-1.6168, 35.1757) -> (-1.6118, 35.1999) construction
  line L290 (-1.6118, 35.1999) -> (-1.66, 35.2303) construction
  line L291 (-1.66, 35.2303) -> (-1.6953, 35.2526) construction
  line L292 (-1.6953, 35.2526) -> (-1.7442, 35.2168) construction
  line L293 (-1.7442, 35.2168) -> (-1.7442, 35.1687) construction
  line L294 (-1.7442, 35.1687) -> (-1.7442, 35.1297) construction
  line L295 (-1.7442, 35.1297) -> (-1.7471, 35.1302) construction
  line L296 (-1.7471, 35.1302) -> (-1.6755, 35.1552) construction
  spline S67 degree 3 poles (-2.9536, 35.2043) (-2.9482, 35.213) (-2.9582, 35.2379) (-2.9758, 35.2596) (-3.003, 35.2931) (-3.0135, 35.2959) (-3.0462, 35.2784) (-3.0973, 35.2511) (-3.0948, 35.2345) (-3.0363, 35.2114) (-2.9725, 35.1862) (-2.9651, 35.1856) (-2.9536, 35.2043) knots 0 0 0 0 1 1 1 2 2 2 3 3 3 4 4 4 4
  line L297 (-2.9536, 35.2043) -> (-2.9482, 35.213) construction
  line L298 (-2.9482, 35.213) -> (-2.9582, 35.2379) construction
  line L299 (-2.9582, 35.2379) -> (-2.9758, 35.2596) construction
  line L300 (-2.9758, 35.2596) -> (-3.003, 35.2931) construction
  line L301 (-3.003, 35.2931) -> (-3.0135, 35.2959) construction
  line L302 (-3.0135, 35.2959) -> (-3.0462, 35.2784) construction
  line L303 (-3.0462, 35.2784) -> (-3.0973, 35.2511) construction
  line L304 (-3.0973, 35.2511) -> (-3.0948, 35.2345) construction
  line L305 (-3.0948, 35.2345) -> (-3.0363, 35.2114) construction
  line L306 (-3.0363, 35.2114) -> (-2.9725, 35.1862) construction
  line L307 (-2.9725, 35.1862) -> (-2.9651, 35.1856) construction
  line L308 (-2.9651, 35.1856) -> (-2.9536, 35.2043) construction
  spline S68 degree 3 poles (-1.4646, 35.2255) (-1.4046, 35.2464) (-1.3915, 35.2838) (-1.438, 35.3017) knots 0 0 0 0 1 1 1 1
  line L309 (-1.4646, 35.2255) -> (-1.4046, 35.2464) construction
  line L310 (-1.4046, 35.2464) -> (-1.3915, 35.2838) construction
  line L311 (-1.3915, 35.2838) -> (-1.438, 35.3017) construction
  spline S69 degree 3 poles (-1.438, 35.3017) (-1.4965, 35.3241) (-1.5687, 35.268) (-1.5404, 35.2222) knots 1 1 1 1 2 2 2 2
  line L312 (-1.438, 35.3017) -> (-1.4965, 35.3241) construction
  line L313 (-1.4965, 35.3241) -> (-1.5687, 35.268) construction
  line L314 (-1.5687, 35.268) -> (-1.5404, 35.2222) construction
  spline S70 degree 3 poles (-1.5404, 35.2222) (-1.5281, 35.2023) (-1.5315, 35.2022) (-1.4646, 35.2255) knots 2 2 2 2 3 3 3 3
  line L315 (-1.5404, 35.2222) -> (-1.5281, 35.2023) construction
  line L316 (-1.5281, 35.2023) -> (-1.5315, 35.2022) construction
  line L317 (-1.5315, 35.2022) -> (-1.4646, 35.2255) construction
  spline S71 degree 3 poles (-3.1591, 35.3145) (-3.1563, 35.3288) (-3.1744, 35.3515) (-3.1993, 35.3648) knots 0 0 0 0 1 1 1 1
  line L318 (-3.1591, 35.3145) -> (-3.1563, 35.3288) construction
  line L319 (-3.1563, 35.3288) -> (-3.1744, 35.3515) construction
  line L320 (-3.1744, 35.3515) -> (-3.1993, 35.3648) construction
  spline S72 degree 3 poles (-3.1993, 35.3648) (-3.2386, 35.3858) (-3.2482, 35.3853) (-3.2726, 35.361) knots 1 1 1 1 2 2 2 2
  line L321 (-3.1993, 35.3648) -> (-3.2386, 35.3858) construction
  line L322 (-3.2386, 35.3858) -> (-3.2482, 35.3853) construction
  line L323 (-3.2482, 35.3853) -> (-3.2726, 35.361) construction
  spline S73 degree 3 poles (-3.2726, 35.361) (-3.2982, 35.3353) (-3.2963, 35.3306) (-3.25, 35.3055) knots 2 2 2 2 3 3 3 3
  line L324 (-3.2726, 35.361) -> (-3.2982, 35.3353) construction
  line L325 (-3.2982, 35.3353) -> (-3.2963, 35.3306) construction
  line L326 (-3.2963, 35.3306) -> (-3.25, 35.3055) construction
  spline S74 degree 3 poles (-3.25, 35.3055) (-3.1924, 35.2744) (-3.1664, 35.2769) (-3.1591, 35.3145) knots 3 3 3 3 4 4 4 4
  line L327 (-3.25, 35.3055) -> (-3.1924, 35.2744) construction
  line L328 (-3.1924, 35.2744) -> (-3.1664, 35.2769) construction
  line L329 (-3.1664, 35.2769) -> (-3.1591, 35.3145) construction
  spline S75 degree 3 poles (-1.2482, 35.3219) (-1.2048, 35.3443) (-1.1988, 35.3541) (-1.2159, 35.3748) (-1.2461, 35.4112) (-1.2988, 35.406) (-1.3211, 35.3645) (-1.3383, 35.3323) (-1.3323, 35.2943) (-1.3101, 35.2943) (-1.3054, 35.2943) (-1.2775, 35.3067) (-1.2482, 35.3219) knots 0 0 0 0 1 1 1 2 2 2 3 3 3 4 4 4 4
  line L330 (-1.2482, 35.3219) -> (-1.2048, 35.3443) construction
  line L331 (-1.2048, 35.3443) -> (-1.1988, 35.3541) construction
  line L332 (-1.1988, 35.3541) -> (-1.2159, 35.3748) construction
  line L333 (-1.2159, 35.3748) -> (-1.2461, 35.4112) construction
  line L334 (-1.2461, 35.4112) -> (-1.2988, 35.406) construction
  line L335 (-1.2988, 35.406) -> (-1.3211, 35.3645) construction
  line L336 (-1.3211, 35.3645) -> (-1.3383, 35.3323) construction
  line L337 (-1.3383, 35.3323) -> (-1.3323, 35.2943) construction
  line L338 (-1.3323, 35.2943) -> (-1.3101, 35.2943) construction
  line L339 (-1.3101, 35.2943) -> (-1.3054, 35.2943) construction
  line L340 (-1.3054, 35.2943) -> (-1.2775, 35.3067) construction
  line L341 (-1.2775, 35.3067) -> (-1.2482, 35.3219) construction
  spline S76 degree 3 poles (-3.3493, 35.4168) (-3.3493, 35.4683) (-3.4164, 35.5091) (-3.4613, 35.4851) (-3.4963, 35.4663) (-3.4958, 35.4646) (-3.4454, 35.4242) (-3.3822, 35.3737) (-3.3493, 35.3711) (-3.3493, 35.4168) knots 0 0 0 0 1 1 1 2 2 2 3 3 3 3
  line L342 (-3.3493, 35.4168) -> (-3.3493, 35.4683) construction
  line L343 (-3.3493, 35.4683) -> (-3.4164, 35.5091) construction
  line L344 (-3.4164, 35.5091) -> (-3.4613, 35.4851) construction
  line L345 (-3.4613, 35.4851) -> (-3.4963, 35.4663) construction
  line L346 (-3.4963, 35.4663) -> (-3.4958, 35.4646) construction
  line L347 (-3.4958, 35.4646) -> (-3.4454, 35.4242) construction
  line L348 (-3.4454, 35.4242) -> (-3.3822, 35.3737) construction
  line L349 (-3.3822, 35.3737) -> (-3.3493, 35.3711) construction
  line L350 (-3.3493, 35.3711) -> (-3.3493, 35.4168) construction
  spline S77 degree 3 poles (-1.0158, 35.4216) (-0.9577, 35.4426) (-0.9602, 35.4628) (-1.0258, 35.5026) (-1.0711, 35.5301) (-1.0756, 35.5298) (-1.1086, 35.4968) (-1.1513, 35.4541) (-1.1398, 35.3734) (-1.0937, 35.3921) (-1.0779, 35.3985) (-1.0429, 35.4118) (-1.0158, 35.4216) knots 0 0 0 0 1 1 1 2 2 2 3 3 3 4 4 4 4
  line L351 (-1.0158, 35.4216) -> (-0.9577, 35.4426) construction
  line L352 (-0.9577, 35.4426) -> (-0.9602, 35.4628) construction
  line L353 (-0.9602, 35.4628) -> (-1.0258, 35.5026) construction
  line L354 (-1.0258, 35.5026) -> (-1.0711, 35.5301) construction
  line L355 (-1.0711, 35.5301) -> (-1.0756, 35.5298) construction
  line L356 (-1.0756, 35.5298) -> (-1.1086, 35.4968) construction
  line L357 (-1.1086, 35.4968) -> (-1.1513, 35.4541) construction
  line L358 (-1.1513, 35.4541) -> (-1.1398, 35.3734) construction
  line L359 (-1.1398, 35.3734) -> (-1.0937, 35.3921) construction
  line L360 (-1.0937, 35.3921) -> (-1.0779, 35.3985) construction
  line L361 (-1.0779, 35.3985) -> (-1.0429, 35.4118) construction
  line L362 (-1.0429, 35.4118) -> (-1.0158, 35.4216) construction
  spline S78 degree 3 poles (-3.536, 35.535) (-3.5243, 35.5655) (-3.5702, 35.6296) (-3.6034, 35.6292) (-3.614, 35.629) (-3.6347, 35.6209) (-3.6492, 35.6111) (-3.6714, 35.5962) (-3.6672, 35.5864) (-3.6227, 35.5498) (-3.5602, 35.4982) (-3.5507, 35.4966) (-3.536, 35.535) knots 0 0 0 0 1 1 1 2 2 2 3 3 3 4 4 4 4
  line L363 (-3.536, 35.535) -> (-3.5243, 35.5655) construction
  line L364 (-3.5243, 35.5655) -> (-3.5702, 35.6296) construction
  line L365 (-3.5702, 35.6296) -> (-3.6034, 35.6292) construction
  line L366 (-3.6034, 35.6292) -> (-3.614, 35.629) construction
  line L367 (-3.614, 35.629) -> (-3.6347, 35.6209) construction
  line L368 (-3.6347, 35.6209) -> (-3.6492, 35.6111) construction
  line L369 (-3.6492, 35.6111) -> (-3.6714, 35.5962) construction
  line L370 (-3.6714, 35.5962) -> (-3.6672, 35.5864) construction
  line L371 (-3.6672, 35.5864) -> (-3.6227, 35.5498) construction
  line L372 (-3.6227, 35.5498) -> (-3.5602, 35.4982) construction
  line L373 (-3.5602, 35.4982) -> (-3.5507, 35.4966) construction
  line L374 (-3.5507, 35.4966) -> (-3.536, 35.535) construction
  spline S79 degree 3 poles (-3.7024, 35.7202) (-3.7021, 35.7511) (-3.7366, 35.7706) (-3.7917, 35.7706) (-3.8389, 35.7706) (-3.8339, 35.7383) (-3.779, 35.6873) (-3.7305, 35.6423) (-3.703, 35.6541) (-3.7024, 35.7202) knots 0 0 0 0 1 1 1 2 2 2 3 3 3 3
  line L375 (-3.7024, 35.7202) -> (-3.7021, 35.7511) construction
  line L376 (-3.7021, 35.7511) -> (-3.7366, 35.7706) construction
  line L377 (-3.7366, 35.7706) -> (-3.7917, 35.7706) construction
  line L378 (-3.7917, 35.7706) -> (-3.8389, 35.7706) construction
  line L379 (-3.8389, 35.7706) -> (-3.8339, 35.7383) construction
  line L380 (-3.8339, 35.7383) -> (-3.779, 35.6873) construction
  line L381 (-3.779, 35.6873) -> (-3.7305, 35.6423) construction
  line L382 (-3.7305, 35.6423) -> (-3.703, 35.6541) construction
  line L383 (-3.703, 35.6541) -> (-3.7024, 35.7202) construction
  spline S80 degree 3 poles (-3.8638, 35.8655) (-3.8562, 35.9048) (-3.8918, 35.947) (-3.9325, 35.947) (-3.9845, 35.947) (-3.991, 35.9122) (-3.9475, 35.8659) knots 0 0 0 0 1 1 1 2 2 2 2
  line L384 (-3.8638, 35.8655) -> (-3.8562, 35.9048) construction
  line L385 (-3.8562, 35.9048) -> (-3.8918, 35.947) construction
  line L386 (-3.8918, 35.947) -> (-3.9325, 35.947) construction
  line L387 (-3.9325, 35.947) -> (-3.9845, 35.947) construction
  line L388 (-3.9845, 35.947) -> (-3.991, 35.9122) construction
  line L389 (-3.991, 35.9122) -> (-3.9475, 35.8659) construction
  spline S81 degree 3 poles (-3.9475, 35.8659) (-3.9031, 35.8187) (-3.8729, 35.8186) (-3.8638, 35.8655) knots 2 2 2 2 3 3 3 3
  line L390 (-3.9475, 35.8659) -> (-3.9031, 35.8187) construction
  line L391 (-3.9031, 35.8187) -> (-3.8729, 35.8186) construction
  line L392 (-3.8729, 35.8186) -> (-3.8638, 35.8655) construction
  line L393 (-3.8638, 35.8655) -> (-3.8638, 35.8655)
  spline S82 degree 3 poles (-3.9985, 36.0786) (-4.0125, 36.1093) (-4.0328, 36.1233) (-4.0633, 36.1233) (-4.1181, 36.1233) (-4.1204, 36.0912) (-4.0701, 36.0273) (-4.0362, 35.9842) (-4.0298, 35.9821) (-4.0053, 36.0066) (-3.9832, 36.0287) (-3.9819, 36.0423) (-3.9985, 36.0786) knots 0 0 0 0 1 1 1 2 2 2 3 3 3 4 4 4 4
  line L394 (-3.9985, 36.0786) -> (-4.0125, 36.1093) construction
  line L395 (-4.0125, 36.1093) -> (-4.0328, 36.1233) construction
  line L396 (-4.0328, 36.1233) -> (-4.0633, 36.1233) construction
  line L397 (-4.0633, 36.1233) -> (-4.1181, 36.1233) construction
  line L398 (-4.1181, 36.1233) -> (-4.1204, 36.0912) construction
  line L399 (-4.1204, 36.0912) -> (-4.0701, 36.0273) construction
  line L400 (-4.0701, 36.0273) -> (-4.0362, 35.9842) construction
  line L401 (-4.0362, 35.9842) -> (-4.0298, 35.9821) construction
  line L402 (-4.0298, 35.9821) -> (-4.0053, 36.0066) construction
  line L403 (-4.0053, 36.0066) -> (-3.9832, 36.0287) construction
  line L404 (-3.9832, 36.0287) -> (-3.9819, 36.0423) construction
  line L405 (-3.9819, 36.0423) -> (-3.9985, 36.0786) construction
  spline S83 degree 3 poles (-4.118, 36.217) (-4.0918, 36.2584) (-4.1252, 36.307) (-4.1846, 36.3141) (-4.2397, 36.3207) (-4.24, 36.3193) (-4.2014, 36.2383) (-4.1701, 36.1726) (-4.1493, 36.1673) (-4.118, 36.217) knots 0 0 0 0 1 1 1 2 2 2 3 3 3 3
  line L406 (-4.118, 36.217) -> (-4.0918, 36.2584) construction
  line L407 (-4.0918, 36.2584) -> (-4.1252, 36.307) construction
  line L408 (-4.1252, 36.307) -> (-4.1846, 36.3141) construction
  line L409 (-4.1846, 36.3141) -> (-4.2397, 36.3207) construction
  line L410 (-4.2397, 36.3207) -> (-4.24, 36.3193) construction
  line L411 (-4.24, 36.3193) -> (-4.2014, 36.2383) construction
  line L412 (-4.2014, 36.2383) -> (-4.1701, 36.1726) construction
  line L413 (-4.1701, 36.1726) -> (-4.1493, 36.1673) construction
  line L414 (-4.1493, 36.1673) -> (-4.118, 36.217) construction
  spline S84 degree 3 poles (-4.2143, 36.4135) (-4.1821, 36.4524) (-4.1996, 36.4999) (-4.2532, 36.5187) (-4.3171, 36.5412) (-4.3272, 36.5265) (-4.2999, 36.451) (-4.2756, 36.3838) (-4.2488, 36.372) (-4.2143, 36.4135) knots 0 0 0 0 1 1 1 2 2 2 3 3 3 3
  line L415 (-4.2143, 36.4135) -> (-4.1821, 36.4524) construction
  line L416 (-4.1821, 36.4524) -> (-4.1996, 36.4999) construction
  line L417 (-4.1996, 36.4999) -> (-4.2532, 36.5187) construction
  line L418 (-4.2532, 36.5187) -> (-4.3171, 36.5412) construction
  line L419 (-4.3171, 36.5412) -> (-4.3272, 36.5265) construction
  line L420 (-4.3272, 36.5265) -> (-4.2999, 36.451) construction
  line L421 (-4.2999, 36.451) -> (-4.2756, 36.3838) construction
  line L422 (-4.2756, 36.3838) -> (-4.2488, 36.372) construction
  line L423 (-4.2488, 36.372) -> (-4.2143, 36.4135) construction
  spline S85 degree 3 poles (-4.2944, 36.6334) (-4.2533, 36.6788) (-4.2841, 36.7407) (-4.3478, 36.7407) (-4.3857, 36.7407) (-4.3907, 36.7347) (-4.381, 36.701) knots 0 0 0 0 1 1 1 2 2 2 2
  line L424 (-4.2944, 36.6334) -> (-4.2533, 36.6788) construction
  line L425 (-4.2533, 36.6788) -> (-4.2841, 36.7407) construction
  line L426 (-4.2841, 36.7407) -> (-4.3478, 36.7407) construction
  line L427 (-4.3478, 36.7407) -> (-4.3857, 36.7407) construction
  line L428 (-4.3857, 36.7407) -> (-4.3907, 36.7347) construction
  line L429 (-4.3907, 36.7347) -> (-4.381, 36.701) construction
  spline S86 degree 3 poles (-4.381, 36.701) (-4.3747, 36.6792) (-4.3657, 36.6474) (-4.361, 36.6305) knots 2 2 2 2 3 3 3 3
  line L430 (-4.381, 36.701) -> (-4.3747, 36.6792) construction
  line L431 (-4.3747, 36.6792) -> (-4.3657, 36.6474) construction
  line L432 (-4.3657, 36.6474) -> (-4.361, 36.6305) construction
  spline S87 degree 3 poles (-4.361, 36.6305) (-4.3499, 36.5907) (-4.3323, 36.5915) (-4.2944, 36.6334) knots 3 3 3 3 4 4 4 4
  line L433 (-4.361, 36.6305) -> (-4.3499, 36.5907) construction
  line L434 (-4.3499, 36.5907) -> (-4.3323, 36.5915) construction
  line L435 (-4.3323, 36.5915) -> (-4.2944, 36.6334) construction
  spline S88 degree 3 poles (-2.0882, 36.7775) (-1.9014, 36.8474) (-1.789, 37.0134) (-1.7898, 37.2185) knots 0 0 0 0 1 1 1 1
  line L436 (-2.0882, 36.7775) -> (-1.9014, 36.8474) construction
  line L437 (-1.9014, 36.8474) -> (-1.789, 37.0134) construction
  line L438 (-1.789, 37.0134) -> (-1.7898, 37.2185) construction
  spline S89 degree 3 poles (-1.7898, 37.2185) (-1.7913, 37.6381) (-2.2636, 37.8512) (-2.5875, 37.5787) knots 1 1 1 1 2 2 2 2
  line L439 (-1.7898, 37.2185) -> (-1.7913, 37.6381) construction
  line L440 (-1.7913, 37.6381) -> (-2.2636, 37.8512) construction
  line L441 (-2.2636, 37.8512) -> (-2.5875, 37.5787) construction
  spline S90 degree 3 poles (-2.5875, 37.5787) (-2.6606, 37.5171) (-2.7057, 37.4385) (-2.7316, 37.3272) knots 2 2 2 2 3 3 3 3
  line L442 (-2.5875, 37.5787) -> (-2.6606, 37.5171) construction
  line L443 (-2.6606, 37.5171) -> (-2.7057, 37.4385) construction
  line L444 (-2.7057, 37.4385) -> (-2.7316, 37.3272) construction
  spline S91 degree 3 poles (-2.7316, 37.3272) (-2.7566, 37.2196) (-2.7363, 37.1028) (-2.6691, 36.9686) knots 3 3 3 3 4 4 4 4
  line L445 (-2.7316, 37.3272) -> (-2.7566, 37.2196) construction
  line L446 (-2.7566, 37.2196) -> (-2.7363, 37.1028) construction
  line L447 (-2.7363, 37.1028) -> (-2.6691, 36.9686) construction
  spline S92 degree 3 poles (-2.6691, 36.9686) (-2.5707, 36.7722) (-2.3215, 36.6902) (-2.0882, 36.7775) knots 4 4 4 4 5 5 5 5
  line L448 (-2.6691, 36.9686) -> (-2.5707, 36.7722) construction
  line L449 (-2.5707, 36.7722) -> (-2.3215, 36.6902) construction
  line L450 (-2.3215, 36.6902) -> (-2.0882, 36.7775) construction
  spline S93 degree 3 poles (-4.3536, 36.8295) (-4.3079, 36.854) (-4.3104, 36.9087) (-4.3587, 36.9426) knots 0 0 0 0 1 1 1 1
  line L451 (-4.3536, 36.8295) -> (-4.3079, 36.854) construction
  line L452 (-4.3079, 36.854) -> (-4.3104, 36.9087) construction
  line L453 (-4.3104, 36.9087) -> (-4.3587, 36.9426) construction
  spline S94 degree 3 poles (-4.3587, 36.9426) (-4.4117, 36.9797) (-4.4254, 36.9772) (-4.4251, 36.9303) knots 1 1 1 1 2 2 2 2
  line L454 (-4.3587, 36.9426) -> (-4.4117, 36.9797) construction
  line L455 (-4.4117, 36.9797) -> (-4.4254, 36.9772) construction
  line L456 (-4.4254, 36.9772) -> (-4.4251, 36.9303) construction
  spline S95 degree 3 poles (-4.4251, 36.9303) (-4.4248, 36.8835) (-4.4069, 36.8113) (-4.3956, 36.8113) (-4.3913, 36.8113) (-4.3724, 36.8195) (-4.3536, 36.8295) knots 2 2 2 2 3 3 3 4 4 4 4
  line L457 (-4.4251, 36.9303) -> (-4.4248, 36.8835) construction
  line L458 (-4.4248, 36.8835) -> (-4.4069, 36.8113) construction
  line L459 (-4.4069, 36.8113) -> (-4.3956, 36.8113) construction
  line L460 (-4.3956, 36.8113) -> (-4.3913, 36.8113) construction
  line L461 (-4.3913, 36.8113) -> (-4.3724, 36.8195) construction
  line L462 (-4.3724, 36.8195) -> (-4.3536, 36.8295) construction
  spline S96 degree 3 poles (-4.3586, 37.1179) (-4.3613, 37.1362) (-4.3814, 37.163) (-4.4033, 37.1774) (-4.4421, 37.2031) (-4.443, 37.2022) (-4.443, 37.1339) (-4.443, 37.0955) (-4.4381, 37.0593) (-4.4322, 37.0534) (-4.4121, 37.0333) (-4.3536, 37.0846) (-4.3586, 37.1179) knots 0 0 0 0 1 1 1 2 2 2 3 3 3 4 4 4 4
  line L463 (-4.3586, 37.1179) -> (-4.3613, 37.1362) construction
  line L464 (-4.3613, 37.1362) -> (-4.3814, 37.163) construction
  line L465 (-4.3814, 37.163) -> (-4.4033, 37.1774) construction
  line L466 (-4.4033, 37.1774) -> (-4.4421, 37.2031) construction
  line L467 (-4.4421, 37.2031) -> (-4.443, 37.2022) construction
  line L468 (-4.443, 37.2022) -> (-4.443, 37.1339) construction
  line L469 (-4.443, 37.1339) -> (-4.443, 37.0955) construction
  line L470 (-4.443, 37.0955) -> (-4.4381, 37.0593) construction
  line L471 (-4.4381, 37.0593) -> (-4.4322, 37.0534) construction
  line L472 (-4.4322, 37.0534) -> (-4.4121, 37.0333) construction
  line L473 (-4.4121, 37.0333) -> (-4.3536, 37.0846) construction
  line L474 (-4.3536, 37.0846) -> (-4.3586, 37.1179) construction
  spline S97 degree 3 poles (-4.3655, 37.3096) (-4.3424, 37.3462) (-4.3684, 37.3989) (-4.414, 37.4079) (-4.4371, 37.4124) (-4.443, 37.3988) (-4.443, 37.3404) (-4.443, 37.282) (-4.4371, 37.2684) (-4.414, 37.273) (-4.398, 37.2761) (-4.3762, 37.2926) (-4.3655, 37.3096) knots 0 0 0 0 1 1 1 2 2 2 3 3 3 4 4 4 4
  line L475 (-4.3655, 37.3096) -> (-4.3424, 37.3462) construction
  line L476 (-4.3424, 37.3462) -> (-4.3684, 37.3989) construction
  line L477 (-4.3684, 37.3989) -> (-4.414, 37.4079) construction
  line L478 (-4.414, 37.4079) -> (-4.4371, 37.4124) construction
  line L479 (-4.4371, 37.4124) -> (-4.443, 37.3988) construction
  line L480 (-4.443, 37.3988) -> (-4.443, 37.3404) construction
  line L481 (-4.443, 37.3404) -> (-4.443, 37.282) construction
  line L482 (-4.443, 37.282) -> (-4.4371, 37.2684) construction
  line L483 (-4.4371, 37.2684) -> (-4.414, 37.273) construction
  line L484 (-4.414, 37.273) -> (-4.398, 37.2761) construction
  line L485 (-4.398, 37.2761) -> (-4.3762, 37.2926) construction
  line L486 (-4.3762, 37.2926) -> (-4.3655, 37.3096) construction
  spline S98 degree 3 poles (-4.3297, 37.5398) (-4.3161, 37.5613) (-4.322, 37.579) (-4.3544, 37.6135) (-4.3855, 37.6466) (-4.4003, 37.6527) (-4.4094, 37.6363) (-4.4207, 37.616) (-4.4319, 37.5271) (-4.4272, 37.4953) (-4.4241, 37.4748) (-4.3492, 37.509) (-4.3297, 37.5398) knots 0 0 0 0 1 1 1 2 2 2 3 3 3 4 4 4 4
  line L487 (-4.3297, 37.5398) -> (-4.3161, 37.5613) construction
  line L488 (-4.3161, 37.5613) -> (-4.322, 37.579) construction